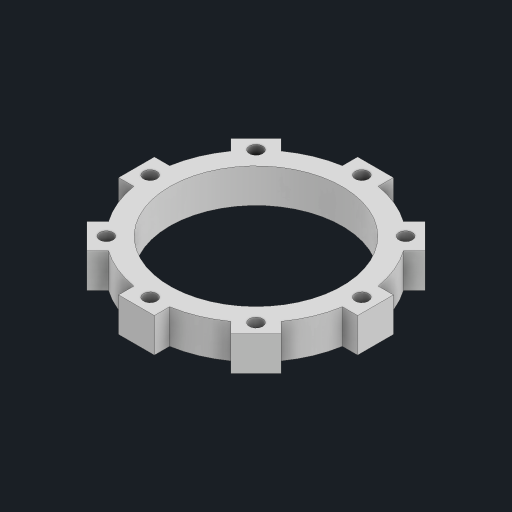
# Autodesk Inventor part: 24vFastener
Saved by Autodesk Inventor 2024 (Build 280153000, 153)
## iProperties
Created: 2023-12-09
Part Number: 24vFastener
Material: Generic
Document SubType Name: Modeling
Designer: 16155
Density: 1 g/cm^3
Appearance: Default
Author: 16155
Autodesk Inventor part; units mm, degrees
ref_plane "YZ Plane" through (0, 0, 0) normal (1, 0, 0) x (0, 1, 0)
ref_plane "XZ Plane" through (0, 0, 0) normal (0, 1, 0) x (-1, 0, 0)
ref_plane "XY Plane" through (0, 0, 0) normal (0, 0, 1) x (1, 0, 0)
sketch "Sketch1" plane through (0, 0, 0) normal (0, 1, 0) x (-1, 0, 0)
  circle A0 centre (0, 0) radius 17
  circle A1 centre (0, 0) radius 13.845
  circle A2 centre (17, 0) radius 1.075
  line L0 (19.2, 2.875) -> (14.8, 2.875)
  line L1 (14.8, 2.875) -> (14.8, -2.875)
  line L2 (14.8, -2.875) -> (19.2, -2.875)
  line L3 (19.2, -2.875) -> (19.2, 2.875)
  line L4 (19.2, 2.875) -> (14.8, -2.875) construction
  line L5 (14.8, 2.875) -> (19.2, -2.875) construction
  circle A3 centre (12.0208, 12.0208) radius 1.075
  line L6 (11.5435, 15.6094) -> (8.4322, 12.4981)
  line L7 (8.4322, 12.4981) -> (12.4981, 8.4322)
  line L8 (12.4981, 8.4322) -> (15.6094, 11.5435)
  line L9 (15.6094, 11.5435) -> (11.5435, 15.6094)
  line L10 (11.5435, 15.6094) -> (12.4981, 8.4322) construction
  line L11 (8.4322, 12.4981) -> (15.6094, 11.5435) construction
  circle A4 centre (0, 17) radius 1.075
  line L12 (-2.875, 19.2) -> (-2.875, 14.8)
  line L13 (-2.875, 14.8) -> (2.875, 14.8)
  line L14 (2.875, 14.8) -> (2.875, 19.2)
  line L15 (2.875, 19.2) -> (-2.875, 19.2)
  line L16 (-2.875, 19.2) -> (2.875, 14.8) construction
  line L17 (-2.875, 14.8) -> (2.875, 19.2) construction
  circle A5 centre (-12.0208, 12.0208) radius 1.075
  line L18 (-15.6094, 11.5435) -> (-12.4981, 8.4322)
  line L19 (-12.4981, 8.4322) -> (-8.4322, 12.4981)
  line L20 (-8.4322, 12.4981) -> (-11.5435, 15.6094)
  line L21 (-11.5435, 15.6094) -> (-15.6094, 11.5435)
  line L22 (-15.6094, 11.5435) -> (-8.4322, 12.4981) construction
  line L23 (-12.4981, 8.4322) -> (-11.5435, 15.6094) construction
  circle A6 centre (-17, 0) radius 1.075
  line L24 (-19.2, -2.875) -> (-14.8, -2.875)
  line L25 (-14.8, -2.875) -> (-14.8, 2.875)
  line L26 (-14.8, 2.875) -> (-19.2, 2.875)
  line L27 (-19.2, 2.875) -> (-19.2, -2.875)
  line L28 (-19.2, -2.875) -> (-14.8, 2.875) construction
  line L29 (-14.8, -2.875) -> (-19.2, 2.875) construction
  circle A7 centre (-12.0208, -12.0208) radius 1.075
  line L30 (-11.5435, -15.6094) -> (-8.4322, -12.4981)
  line L31 (-8.4322, -12.4981) -> (-12.4981, -8.4322)
  line L32 (-12.4981, -8.4322) -> (-15.6094, -11.5435)
  line L33 (-15.6094, -11.5435) -> (-11.5435, -15.6094)
  line L34 (-11.5435, -15.6094) -> (-12.4981, -8.4322) construction
  line L35 (-8.4322, -12.4981) -> (-15.6094, -11.5435) construction
  circle A8 centre (0, -17) radius 1.075
  line L36 (2.875, -19.2) -> (2.875, -14.8)
  line L37 (2.875, -14.8) -> (-2.875, -14.8)
  line L38 (-2.875, -14.8) -> (-2.875, -19.2)
  line L39 (-2.875, -19.2) -> (2.875, -19.2)
  line L40 (2.875, -19.2) -> (-2.875, -14.8) construction
  line L41 (2.875, -14.8) -> (-2.875, -19.2) construction
  circle A9 centre (12.0208, -12.0208) radius 1.075
  line L42 (15.6094, -11.5435) -> (12.4981, -8.4322)
  line L43 (12.4981, -8.4322) -> (8.4322, -12.4981)
  line L44 (8.4322, -12.4981) -> (11.5435, -15.6094)
  line L45 (11.5435, -15.6094) -> (15.6094, -11.5435)
  line L46 (15.6094, -11.5435) -> (8.4322, -12.4981) construction
  line L47 (12.4981, -8.4322) -> (11.5435, -15.6094) construction
  point P0 (16.7551, 2.875)
  point P1 (13.8806, 9.8147)
  point P2 (9.8147, 13.8806)
  point P3 (2.875, 16.7551)
  point P4 (-2.875, 16.7551)
  point P5 (-9.8147, 13.8806)
  point P6 (-13.8806, 9.8147)
  point P7 (-16.7551, 2.875)
  point P8 (-16.7551, -2.875)
  point P9 (-13.8806, -9.8147)
  point P10 (-9.8147, -13.8806)
  point P11 (-2.875, -16.7551)
  point P12 (2.875, -16.7551)
  point P13 (9.8147, -13.8806)
  point P14 (13.8806, -9.8147)
  point P15 (16.7551, -2.875)
  dimension "d0" = 34
  dimension "d1" = 27.69
  dimension "d2" = 5.75
  dimension "d3" = 2.15
  dimension "d4" = 4.4
  dimension "d7" = 360
  constraints: 96 end point, 10 centre point, 2 coincident, 2 midpoint, 2 parallel, 2 point on circle, 1 horizontal, 1 perpendicular, 105 other
  measures "d0" diameter of A0
  measures "d1" diameter of A1
  measures "d2" distance of L2.end L0.start
  measures "d3" diameter of A2
  measures "d4" distance of L1.end L2.end
extrude "Extrusion1" add sketch "Sketch1" along normal blind 5.5 contours A2 A0 L2 L1 L0 | A0 L0 L3 L2 A2 | L0 L1 L2 A0 L42 L43 L44 L36 L37 L38 L30 L31 L32 L24 L25 L26 L18 L19 L20 L12 L13 L14 L6 L7 L8 | L8 L7 L6 A0 A3 | A0 A3 L6 L9 L8 | L42 L45 L44 A0 A9 | A0 A9 L44 L43 L42 | L14 L13 L12 A0 A4 | A0 A4 L12 L15 L14 | L36 L39 L38 A0 A8 | A0 A8 L38 L37 L36 | L20 L19 L18 A0 A5 | A0 A5 L18 L21 L20 | L30 L33 L32 A0 A7 | A0 A7 L32 L31 L30 | L26 L25 L24 A0 A6 | A0 A6 L24 L27 L26
body "Solid1"
